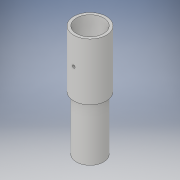
# Autodesk Inventor part: outer_chamber_v4
Saved by Autodesk Inventor 2019 (Build 230136000, 136)
## iProperties
Created: 2021-01-22
Part Number: outer_chamber_v4
Material: Generic
Document SubType Name: Modeling
Designer: wilson
Density: 1 g/cm^3
Appearance: Default
Author: wilson
Autodesk Inventor part; units mm, degrees
ref_plane "YZ Plane" through (0, 0, 0) normal (1, 0, 0) x (0, 1, 0)
ref_plane "XZ Plane" through (0, 0, 0) normal (0, 1, 0) x (-1, 0, 0)
ref_plane "XY Plane" through (0, 0, 0) normal (0, 0, 1) x (1, 0, 0)
sketch "Sketch1" plane through (0, 0, 0) normal (0, 1, 0) x (-1, 0, 0)
  circle A0 centre (0, 0) radius 6
  dimension "d0" = 12
  constraints: 1 centre point, 1 coincident
  measures "d0" diameter of A0
extrude "Extrusion1" add sketch "Sketch1" against normal blind 10
sketch "Sketch2" plane through (0, 0, 0) normal (0, 1, 0) x (1, 0, 0)
  point P0 (0, 0)
  point P1 (0, 0)
  constraints: 1 coincident
hole "Hole1" at (0, 0, 0) direction (0, -1, 0) diameter 10 depth 39 tip angle 118
sketch "Sketch3" plane through (0, 0, 0) normal (0, 1, 0) x (1, 0, 0)
  point P0 (0, 0)
sketch "Sketch4" plane through (0, 0, 0) normal (0, 1, 0) x (1, 0, 0)
  point P0 (0, 0)
sketch "Sketch5" plane through (0, 0, 0) normal (0, 1, 0) x (1, 0, 0)
  line L0 (0, -4.4606) -> (0.5, -4.4606)
  line L1 (0.5, -4.4606) -> (0.5, -6.4217)
  line L2 (0.5, -6.4217) -> (0, -6.4217)
  line L3 (0, -6.4217) -> (0, -4.4606)
  point P0 (0, 0)
  dimension "d10" = 0.5
  constraints: 8 end point, 2 parallel, 1 horizontal, 1 perpendicular
  measures "d10" distance of L1.end L2.end
revolve "Revolution1" cut sketch "Sketch5" angle 360 about axis through (0, 0, 6.4217) along (0, 0, -1)
sketch "Sketch6" plane through (0, 0, 0) normal (0, 1, 0) x (1, 0, 0)
  circle A0 centre (0, 0) radius 6
  constraints: 1 centre point, 1 coincident
extrude "Extrusion2" add sketch "Sketch6" along normal blind 10
sketch "Sketch7" plane through (0, 10, 0) normal (0, 1, 0) x (1, 0, 0)
  point P0 (0, 0)
  point P1 (0, 0)
  constraints: 1 coincident
hole "Hole2" at (0, 10, 0) direction (0, -1, 0) diameter 10 depth 39 tip angle 118
pattern_circular "Circular Pattern1" count 2 over 360 about axis through (0, 0, -10) along (0, 0, 1) of "Revolution1"
pattern_circular "Circular Pattern2" count 2 over 360 about axis through (0, -10, 0) along (0, 1, 0) of "Revolution1", "Circular Pattern1"
sketch "Sketch8" plane through (0, -10, 0) normal (0, -1, 0) x (1, 0, 0)
  circle A0 centre (0, 0) radius 6
  constraints: 1 centre point, 1 coincident
extrude "Extrusion3" add sketch "Sketch8" along normal blind 1
hole "Hole3" at (0, 0, 0) direction (0, -1, 0) diameter 8 depth 39 tip angle 118
sketch "Sketch9" plane through (0, -11, 0) normal (0, -1, 0) x (1, 0, 0)
  circle A0 centre (0, 0) radius 5
  dimension "d36" = 10
  constraints: 1 centre point, 1 coincident
  measures "d36" diameter of A0
extrude "Extrusion4" add sketch "Sketch9" along normal blind 20
sketch "Sketch10" plane through (0, -31, 0) normal (0, -1, 0) x (1, 0, 0)
  point P0 (0, 0)
  point P1 (0, 0)
  constraints: 1 coincident
hole "Hole4" at (0, -31, 0) direction (0, 1, 0) diameter 8 depth 391.2125 tip angle 118
body "Solid1"
